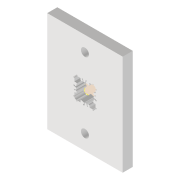
# Autodesk Inventor part: Soporte Pistón
Saved by Autodesk Inventor 2021 (Build 250183000, 183)
## iProperties
Created: 2021-05-02
Part Number: Soporte Pistón
Material: Generic
Document SubType Name: Modeling
Designer: maaro
Density: 1 g/cm^3
Appearance: Default
Author: maaro
Autodesk Inventor part; units mm, degrees
ref_plane "YZ Plane" through (0, 0, 0) normal (1, 0, 0) x (0, 1, 0)
ref_plane "XZ Plane" through (0, 0, 0) normal (0, 1, 0) x (-1, 0, 0)
ref_plane "XY Plane" through (0, 0, 0) normal (0, 0, 1) x (1, 0, 0)
ref_plane "Work Plane1" through (0, 0, 0) normal (0, 0, 1) x (1, 0, 0)
sketch "Sketch1" plane through (0, 0, 0) normal (0, 0, 1) x (1, 0, 0)
  circle A0 centre (0, 52.9) radius 8 projected
  line L0 (-75, -117.1) -> (75, -117.1) projected
  line L1 (75, -117.1) -> (75, 82.9) projected
  line L2 (75, 82.9) -> (-75, 82.9) projected
  line L3 (-75, 82.9) -> (-75, -117.1) projected
  circle A1 centre (0, -87.1) radius 8 projected
  circle A2 centre (0, -16.8) radius 16
  line L4 (0.031, -34.3) -> (-1.6246, -39.8894)
  line L5 (-1.6246, -39.8894) -> (-3.8779, -39.222)
  line L6 (-3.8779, -39.222) -> (-3.5087, -37.9755)
  line L7 (-3.5087, -37.9755) -> (-2.8854, -38.1601)
  line L8 (-2.8854, -38.1601) -> (-1.8914, -34.8042)
  line L9 (-1.8914, -34.8042) -> (-8.2196, -32.9297)
  line L10 (-8.2196, -32.9297) -> (-9.2136, -36.2856)
  line L11 (-9.2136, -36.2856) -> (-8.5904, -36.4702)
  line L12 (-8.5904, -36.4702) -> (-8.9843, -37.8)
  line L13 (-8.9843, -37.8) -> (-15.25, -37.8)
  line L14 (-15.25, -37.8) -> (-15.25, -39.8)
  line L15 (-15.25, -39.8) -> (-17.25, -39.8)
  line L16 (-17.25, -39.8) -> (-17.25, -37.8)
  arc A3 (-21, -34.05) -> (-17.25, -37.8) centre (-17.25, -34.05) ccw
  line L17 (-21, -34.05) -> (-23, -34.05)
  line L18 (-23, -34.05) -> (-23, -32.05)
  line L19 (-23, -32.05) -> (-21, -32.05)
  line L20 (-21, -32.05) -> (-21, -26.253)
  line L21 (-21, -26.253) -> (-19.5478, -25.71)
  arc A4 (-19.5478, -25.71) -> (-20.5984, -22.9) centre (-18.6632, -23.7779) ccw
  line L22 (-20.5984, -22.9) -> (-21.4365, -23.2134)
  line L23 (-21.4365, -23.2134) -> (-22.1807, -21.2229)
  line L24 (-22.1807, -21.2229) -> (-17.3057, -19.4003)
  arc A5 (-17.5, -16.831) -> (-17.3057, -19.4003) centre (0, -16.8) ccw
  line L25 (-17.5, -16.831) -> (-23.0894, -15.1754)
  line L26 (-23.0894, -15.1754) -> (-22.422, -12.9221)
  line L27 (-22.422, -12.9221) -> (-21.1755, -13.2913)
  line L28 (-21.1755, -13.2913) -> (-21.3601, -13.9146)
  line L29 (-21.3601, -13.9146) -> (-18.0042, -14.9086)
  line L30 (-18.0042, -14.9086) -> (-16.1297, -8.5804)
  line L31 (-16.1297, -8.5804) -> (-19.4856, -7.5864)
  line L32 (-19.4856, -7.5864) -> (-19.6702, -8.2096)
  line L33 (-19.6702, -8.2096) -> (-21, -7.8157)
  line L34 (-21, -7.8157) -> (-21, -1.55)
  line L35 (-21, -1.55) -> (-23, -1.55)
  line L36 (-23, -1.55) -> (-23, 0.45)
  line L37 (-23, 0.45) -> (-21, 0.45)
  arc A6 (-17.25, 4.2) -> (-21, 0.45) centre (-17.25, 0.45) ccw
  line L38 (-17.25, 4.2) -> (-17.25, 6.2)
  line L39 (-17.25, 6.2) -> (-15.25, 6.2)
  line L40 (-15.25, 6.2) -> (-15.25, 4.2)
  line L41 (-15.25, 4.2) -> (-9.453, 4.2)
  line L42 (-9.453, 4.2) -> (-8.91, 2.7478)
  arc A7 (-8.91, 2.7478) -> (-6.1, 3.7984) centre (-6.9779, 1.8632) ccw
  line L43 (-6.1, 3.7984) -> (-6.4134, 4.6365)
  line L44 (-6.4134, 4.6365) -> (-4.4229, 5.3807)
  line L45 (-4.4229, 5.3807) -> (-2.6003, 0.5057)
  arc A8 (-0.031, 0.7) -> (-2.6003, 0.5057) centre (0, -16.8) ccw
  line L46 (-0.031, 0.7) -> (1.6246, 6.2894)
  line L47 (1.6246, 6.2894) -> (3.8779, 5.622)
  line L48 (3.8779, 5.622) -> (3.5087, 4.3755)
  line L49 (3.5087, 4.3755) -> (2.8854, 4.5601)
  line L50 (2.8854, 4.5601) -> (1.8914, 1.2042)
  line L51 (1.8914, 1.2042) -> (8.2196, -0.6703)
  line L52 (8.2196, -0.6703) -> (9.2136, 2.6856)
  line L53 (9.2136, 2.6856) -> (8.5904, 2.8702)
  line L54 (8.5904, 2.8702) -> (8.9843, 4.2)
  line L55 (8.9843, 4.2) -> (15.25, 4.2)
  line L56 (15.25, 4.2) -> (15.25, 6.2)
  line L57 (15.25, 6.2) -> (17.25, 6.2)
  line L58 (17.25, 6.2) -> (17.25, 4.2)
  arc A9 (21, 0.45) -> (17.25, 4.2) centre (17.25, 0.45) ccw
  line L59 (21, 0.45) -> (23, 0.45)
  line L60 (23, 0.45) -> (23, -1.55)
  line L61 (23, -1.55) -> (21, -1.55)
  line L62 (21, -1.55) -> (21, -7.347)
  line L63 (21, -7.347) -> (19.5478, -7.89)
  arc A10 (19.5478, -7.89) -> (20.5984, -10.7) centre (18.6632, -9.8221) ccw
  line L64 (20.5984, -10.7) -> (21.4365, -10.3866)
  line L65 (21.4365, -10.3866) -> (22.1807, -12.3771)
  line L66 (22.1807, -12.3771) -> (17.3057, -14.1997)
  arc A11 (17.5, -16.769) -> (17.3057, -14.1997) centre (0, -16.8) ccw
  line L67 (17.5, -16.769) -> (23.0894, -18.4246)
  line L68 (23.0894, -18.4246) -> (22.422, -20.6779)
  line L69 (22.422, -20.6779) -> (21.1755, -20.3087)
  line L70 (21.1755, -20.3087) -> (21.3601, -19.6854)
  line L71 (21.3601, -19.6854) -> (18.0042, -18.6914)
  line L72 (18.0042, -18.6914) -> (16.1297, -25.0196)
  line L73 (16.1297, -25.0196) -> (19.4856, -26.0136)
  line L74 (19.4856, -26.0136) -> (19.6702, -25.3904)
  line L75 (19.6702, -25.3904) -> (21, -25.7843)
  line L76 (21, -25.7843) -> (21, -32.05)
  line L77 (21, -32.05) -> (23, -32.05)
  line L78 (23, -32.05) -> (23, -34.05)
  line L79 (23, -34.05) -> (21, -34.05)
  arc A12 (17.25, -37.8) -> (21, -34.05) centre (17.25, -34.05) ccw
  line L80 (17.25, -37.8) -> (17.25, -39.8)
  line L81 (17.25, -39.8) -> (15.25, -39.8)
  line L82 (15.25, -39.8) -> (15.25, -37.8)
  line L83 (15.25, -37.8) -> (9.453, -37.8)
  line L84 (9.453, -37.8) -> (8.91, -36.3478)
  arc A13 (8.91, -36.3478) -> (6.1, -37.3984) centre (6.9779, -35.4632) ccw
  line L85 (6.1, -37.3984) -> (6.4134, -38.2365)
  line L86 (6.4134, -38.2365) -> (4.4229, -38.9807)
  line L87 (4.4229, -38.9807) -> (2.6003, -34.1057)
  arc A14 (0.031, -34.3) -> (2.6003, -34.1057) centre (0, -16.8) ccw
  constraints: 168 end point, 24 point on circle, 16 horizontal, 16 vertical, 13 centre point, 174 other
extrude "Extrusion1" add sketch "Sketch1" along normal blind 20 contours L3 L2 L1 L0
body "Solid1"
